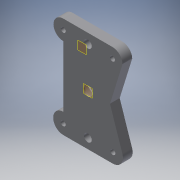
# Autodesk Inventor part: Endstop
Saved by Autodesk Inventor 2016 (Build 200138000, 138)
## iProperties
Created: 2016-04-20
Part Number: Endstop
Material: Generic
Document SubType Name: Modeling
Designer: Scott
Density: 1 g/cm^3
Appearance: Default
Author: Scott
Autodesk Inventor part; units mm, degrees
ref_plane "YZ Plane" through (0, 0, 0) normal (1, 0, 0) x (0, 1, 0)
ref_plane "XZ Plane" through (0, 0, 0) normal (0, 1, 0) x (-1, 0, 0)
ref_plane "XY Plane" through (0, 0, 0) normal (0, 0, 1) x (1, 0, 0)
ref_plane "Work Plane1" through (-43.5338, -0.5007, 1.2381) normal (0, 0, 1) x (1, 0, 0)
ref_plane "Work Plane2" through (-43.5338, -42.3785, -4.7563) normal (0, 0, 1) x (1, 0, 0)
sketch "Sketch1" plane through (-43.5338, -42.3785, -4.7563) normal (0, 0, 1) x (1, 0, 0)
  circle A0 centre (0, 41.8778) radius 4 projected
  circle A1 centre (0, 0) radius 4 projected
  circle A2 centre (0, -41.8778) radius 4 projected
  circle A3 centre (-25.4, 41.8778) radius 2.54
  circle A4 centre (-25.3932, -41.7189) radius 2.54
  circle A5 centre (25.3979, 41.5493) radius 2.54
  circle A6 centre (25.8472, -41.7284) radius 2.54
  arc A7 (-24.8901, 51.9352) -> (-25.3932, 31.8075) centre (-25.4, 41.8778) ccw
  arc A8 (-25.3932, -31.3333) -> (-25.3932, -52.1046) centre (-25.3932, -41.7189) ccw
  arc A9 (25.4047, -52.1046) -> (35.6974, -38.4367) centre (25.8472, -41.7284) ccw
  arc A10 (35.7786, 41.8776) -> (25.3979, 51.9352) centre (25.3979, 41.5493) ccw
  line L0 (-24.8901, 51.9352) -> (25.3979, 51.9352)
  line L1 (35.7786, 41.8776) -> (22.8529, -0.0002)
  line L2 (22.8529, -0.0002) -> (35.6974, -38.4367)
  line L3 (25.4047, -52.1046) -> (-25.3932, -52.1046)
  line L4 (-25.3932, -31.3333) -> (-25.3932, 31.8075)
  point P0 (43.5338, 42.3785)
  dimension "d0" = 5.08
  dimension "d1" = 25.4
  dimension "d2" = 5.08
  dimension "d3" = 5.08
  dimension "d4" = 5.08
  dimension "d5" = 25.4
  constraints: 10 end point, 8 centre point, 8 point on circle, 4 coincident, 3 tangent, 1 perpendicular
  measures "d0" diameter of A3
  measures "d1" distance of A3.centre A0.centre
  measures "d2" diameter of A4
  measures "d3" diameter of A5
  measures "d4" diameter of A6
  measures "d5" distance of A5.centre A0.centre
extrude "Extrusion1" add sketch "Sketch1" against normal blind 10
sketch "Sketch2" plane through (-43.5338, -42.3785, -14.7563) normal (0, 0, -1) x (-1, 0, 0)
  circle A0 centre (0, -41.8778) radius 4 projected
  circle A1 centre (0, 0) radius 4 projected
  circle A2 centre (0, 41.8778) radius 4 projected
  circle A3 centre (-25.8472, -41.7284) radius 2.54 projected
  circle A4 centre (-25.3979, 41.5493) radius 2.54 projected
  circle A5 centre (25.3932, -41.7189) radius 2.54 projected
  circle A6 centre (25.4, 41.8778) radius 2.54 projected
  arc A7 (25.3932, 31.8075) -> (24.8901, 51.9352) centre (25.4, 41.8778) ccw projected
  line L0 (25.3932, 31.8075) -> (25.3932, -31.3333) projected
  arc A8 (25.3932, -52.1046) -> (25.3932, -31.3333) centre (25.3932, -41.7189) ccw projected
  line L1 (25.3932, -52.1046) -> (-25.4047, -52.1046) projected
  arc A9 (-35.6974, -38.4367) -> (-25.4047, -52.1046) centre (-25.8472, -41.7284) ccw projected
  line L2 (-35.6974, -38.4367) -> (-22.8529, -0.0002) projected
  line L3 (-22.8529, -0.0002) -> (-35.7786, 41.8776) projected
  arc A10 (-25.3979, 51.9352) -> (-35.7786, 41.8776) centre (-25.3979, 41.5493) ccw projected
  line L4 (-25.3979, 51.9352) -> (24.8901, 51.9352) projected
  circle A11 centre (0, 0) radius 11
  point P0 (-43.5338, 42.3785)
  dimension "d8" = 22
  constraints: 1 centre point, 1 coincident
  measures "d8" diameter of A11
extrude "Extrusion2" cut sketch "Sketch2" against normal blind 8 contours A11
sketch "Sketch3" plane through (-43.5338, -42.3785, -4.7563) normal (0, 0, 1) x (1, 0, 0)
  circle A0 centre (0, 0) radius 5
  point P0 (43.5338, 42.3785)
  dimension "d11" = 10
  constraints: 1 centre point
  measures "d11" diameter of A0
extrude "Extrusion3" cut sketch "Sketch3" against normal blind 8
sketch "Sketch4" plane through (-43.5338, -42.3785, -14.7563) normal (0, 0, -1) x (-1, 0, 0)
  circle A0 centre (0, 0) radius 11 projected
  circle A1 centre (0, -41.8778) radius 4 projected
  circle A2 centre (0, 41.8778) radius 4 projected
  circle A3 centre (-25.8472, -41.7284) radius 2.54 projected
  circle A4 centre (-25.3979, 41.5493) radius 2.54 projected
  circle A5 centre (25.3932, -41.7189) radius 2.54 projected
  circle A6 centre (25.4, 41.8778) radius 2.54 projected
  arc A7 (25.3932, 31.8075) -> (24.8901, 51.9352) centre (25.4, 41.8778) ccw projected
  line L0 (24.8901, 51.9352) -> (-25.3979, 51.9352) projected
  arc A8 (-25.3979, 51.9352) -> (-35.7786, 41.8776) centre (-25.3979, 41.5493) ccw projected
  line L1 (-35.7786, 41.8776) -> (-22.8529, -0.0002) projected
  line L2 (-22.8529, -0.0002) -> (-35.6974, -38.4367) projected
  arc A9 (-35.6974, -38.4367) -> (-25.4047, -52.1046) centre (-25.8472, -41.7284) ccw projected
  line L3 (-25.4047, -52.1046) -> (25.3932, -52.1046) projected
  arc A10 (25.3932, -52.1046) -> (25.3932, -31.3333) centre (25.3932, -41.7189) ccw projected
  line L4 (25.3932, -31.3333) -> (25.3932, 31.8075) projected
  line L5 (-19.5055, 3.4405) -> (-29.2362, 34.9666)
  arc A11 (-26.1883, -47.8914) -> (-25.5061, -47.8914) centre (-25.8472, -41.7284) ccw
  line L6 (-30.2853, -35.5342) -> (-19.5947, -3.5433)
  circle A12 centre (0, 41.8778) radius 4 projected
  arc A13 (-29.2362, 34.9666) -> (-20.9299, 47.722) centre (-25.3979, 41.5493) ccw
  arc A14 (-21.366, -47.8914) -> (-30.2853, -35.5342) centre (-25.8472, -41.7284) ccw
  arc A15 (21.18, -35.3697) -> (20.925, -47.8914) centre (25.3932, -41.7189) ccw
  line L7 (-15.0962, 3.4405) -> (-19.5055, 3.4405)
  line L8 (-19.5947, -3.5433) -> (-15.0962, -3.5433)
  line L9 (21.18, 4.0176) -> (15.57, 4.0176)
  line L10 (15.6848, -3.5433) -> (21.18, -3.5433)
  line L11 (23.5004, 3.4405) -> (23.5004, 4.0176)
  line L12 (-2.4388, 15.894) -> (-2.4388, 33.1315)
  line L13 (1.6137, 32.9424) -> (1.6137, 15.9988)
  line L14 (-2.4388, -15.894) -> (-2.4388, -33.1315)
  line L15 (1.6137, -32.9424) -> (1.6137, -15.9988)
  line L16 (21.18, 35.533) -> (21.18, 4.0176)
  line L17 (21.18, -3.5433) -> (21.18, -37.208)
  arc A16 (20.5102, 47.722) -> (21.18, 35.533) centre (25.4, 41.8778) ccw
  line L18 (-20.9299, 47.722) -> (-6.9492, 47.722)
  line L19 (6.9492, 47.722) -> (20.5102, 47.722)
  arc A17 (15.57, 4.0176) -> (0.9078, 16.0544) centre (0, 0) ccw
  arc A18 (-2.4388, 15.894) -> (-15.7076, 3.4405) centre (0, 0) ccw
  arc A19 (-6.9492, 47.722) -> (-2.4388, 33.1315) centre (0, 41.8778) ccw
  arc A20 (1.6137, 32.9424) -> (6.9492, 47.722) centre (0, 41.8778) ccw
  arc A21 (-15.6848, -3.5433) -> (-1.8329, -15.9752) centre (0, 0) ccw
  arc A22 (0.9945, -16.0492) -> (15.6848, -3.5433) centre (0, 0) ccw
  arc A23 (-2.0453, -33.0312) -> (-6.8032, -47.8914) centre (0, -41.8778) ccw
  arc A24 (6.8032, -47.8914) -> (1.1925, -32.8765) centre (0, -41.8778) ccw
  line L20 (20.925, -47.8914) -> (6.8032, -47.8914)
  line L21 (-6.8032, -47.8914) -> (-21.366, -47.8914)
  point P0 (-43.5338, 42.3785)
  point P1 (18.8824, 0.2371)
  point P2 (-0.4126, 23.807)
  point P3 (-0.4126, -23.9098)
  dimension "d16" = 5.08
  dimension "d17" = 5.08
  dimension "d18" = 5.08
  dimension "d20" = 5.08
  constraints: 34 end point, 31 point on circle, 13 centre point, 5 point on line, 4 parallel, 2 horizontal
  measures "d16" radial gap between concentric circles of A4 A13
  measures "d17" radial gap between concentric circles of A3 A14
  measures "d18" radial gap between concentric circles of A5 A15
  measures "d20" radial gap between concentric circles of A6 A16
extrude "Extrusion4" cut sketch "Sketch4" against normal blind 6.5 contours L5 A13 L18 A19 L12 A18 L7 | L6 L8 A21 L14 A23 L21 A14 | A15 L20 A24 L15 A22 L10 L17 | L9 A17 L13 A20 L19 A16 L16
body "Solid1"
